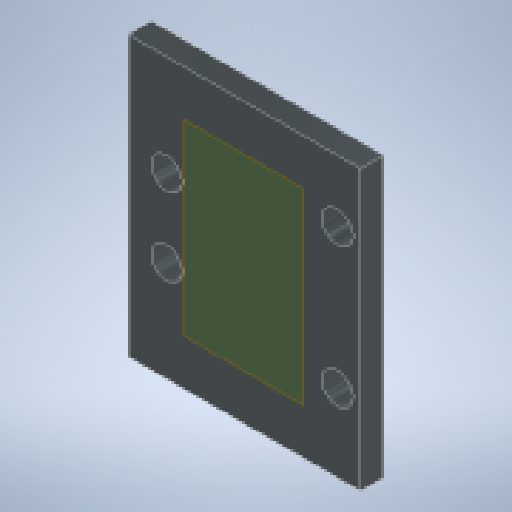
# Autodesk Inventor part: class2
Saved by Autodesk Inventor 2024.2 (Build 282272000, 272)
## iProperties
Created: 2024-07-24
Part Number: class2
Material: Iron, Ductile
Document SubType Name: Modeling
Designer: eamon
Density: 7.15 g/cm^3
Appearance: Iron Gray
Author: eamon
Autodesk Inventor part; units mm, degrees
ref_plane "YZ Plane" through (0, 0, 0) normal (1, 0, 0) x (0, 1, 0)
ref_plane "XZ Plane" through (0, 0, 0) normal (0, 1, 0) x (-1, 0, 0)
ref_plane "XY Plane" through (0, 0, 0) normal (0, 0, 1) x (1, 0, 0)
ref_plane "Work Plane1" through (163.8219, -116.7983, -107.5891) normal (0, 0, -1) x (-1, 0, 0)
sketch "Sketch1" plane through (163.8219, -116.7983, -107.5891) normal (0, 0, -1) x (-1, 0, 0)
  line L0 (-95.25, 114.3) -> (95.25, 114.3)
  line L1 (95.25, 114.3) -> (95.25, -114.3)
  line L2 (95.25, -114.3) -> (-95.25, -114.3)
  line L3 (-95.25, -114.3) -> (-95.25, 114.3)
  line L4 (-95.25, 114.3) -> (95.25, -114.3) construction
  line L5 (95.25, 114.3) -> (-95.25, -114.3) construction
  arc A0 (44.45, 50.8) -> (25.4, 69.85) centre (25.4, 50.8) ccw construction
  line L6 (25.4, 69.85) -> (-25.4, 69.85) construction
  arc A1 (-25.4, 69.85) -> (-44.45, 50.8) centre (-25.4, 50.8) ccw construction
  line L7 (-44.45, 50.8) -> (-44.45, -50.8) construction
  arc A2 (-44.45, -50.8) -> (-25.4, -69.85) centre (-25.4, -50.8) ccw construction
  line L8 (-25.4, -69.85) -> (25.4, -69.85) construction
  arc A3 (25.4, -69.85) -> (44.45, -50.8) centre (25.4, -50.8) ccw construction
  line L9 (44.45, -50.8) -> (44.45, 50.8) construction
  line L10 (38.1, 50.8) -> (38.1, -50.8) construction
  arc A4 (25.4, -63.5) -> (38.1, -50.8) centre (25.4, -50.8) ccw construction
  line L11 (25.4, -63.5) -> (-25.4, -63.5) construction
  arc A5 (-38.1, -50.8) -> (-25.4, -63.5) centre (-25.4, -50.8) ccw construction
  line L12 (-38.1, -50.8) -> (-38.1, 50.8) construction
  arc A6 (-25.4, 63.5) -> (-38.1, 50.8) centre (-25.4, 50.8) ccw construction
  line L13 (-25.4, 63.5) -> (25.4, 63.5) construction
  arc A7 (38.1, 50.8) -> (25.4, 63.5) centre (25.4, 50.8) ccw construction
  circle A8 centre (-76.2, 63.5) radius 12.7
  circle A9 centre (-76.2, -50.8) radius 12.7
  circle A10 centre (63.5, 31.75) radius 12.7
  circle A11 centre (63.5, -31.75) radius 12.7
  point P0 (163.8219, 116.7983)
  point P1 (0, 0)
  point P2 (0, 63.5)
  point P3 (38.1, 0)
  dimension "d0" = 228.6
  dimension "d1" = 190.5
  dimension "d2" = 25.4
  dimension "d3" = 19.05
  dimension "d4" = 114.3
  dimension "d5" = 63.5
  dimension "d6" = 31.75
  dimension "d7" = 63.5
  dimension "d8" = 82.55
  constraints: 12 end point, 4 centre point, 4 midpoint, 3 equal radius, 3 vertical alignment, 2 parallel, 1 horizontal, 1 horizontal alignment, 1 perpendicular
  measures "d0" distance of L0.end L1.end
  measures "d1" distance of L0.start L0.end
  measures "d2" diameter of A8
  measures "d3" distance from line of L3 A8.centre
  measures "d4" distance of A9.centre A8.centre
  measures "d5" distance from line of L2 A9.centre
  measures "d6" distance from line of L1 A10.centre
  measures "d7" distance of A11.centre A10.centre
  measures "d8" distance from line of L0 A10.centre
extrude "Extrusion1" add sketch "Sketch1" along normal blind 19.05
body "Solid1"
